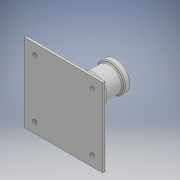
# Autodesk Inventor part: 相机
Saved by Autodesk Inventor 2017 (Build 210142000, 142)
## iProperties
Part Number: 相机
Material: 常规
Document SubType Name: Modeling
Designer: Administrator
Density: 1 g/cm^3
Appearance: 默认
Author: Administrator
Autodesk Inventor part; units mm, degrees
ref_plane "YZ Plane" through (0, 0, 0) normal (1, 0, 0) x (0, 1, 0)
ref_plane "XZ Plane" through (0, 0, 0) normal (0, 1, 0) x (-1, 0, 0)
ref_plane "XY Plane" through (0, 0, 0) normal (0, 0, 1) x (1, 0, 0)
sketch "草图1" plane through (0, 0, 0) normal (0, 1, 0) x (-1, 0, 0)
  line L0 (19, 19) -> (19, -19)
  line L1 (19, -19) -> (-19, -19)
  line L2 (-19, -19) -> (-19, 19)
  line L3 (-19, 19) -> (19, 19)
  line L4 (19, 19) -> (-19, -19) construction
  line L5 (19, -19) -> (-19, 19) construction
  line L6 (14, 14) -> (-14, -14) construction
  line L7 (14, -14) -> (-14, 14) construction
  circle A0 centre (14, 14) radius 1
  circle A1 centre (14, -14) radius 1
  circle A2 centre (-14, -14) radius 1
  circle A3 centre (-14, 14) radius 1
  line L8 (8, 8) -> (-8, -8) construction
  line L9 (8, -8) -> (-8, 8) construction
  point P0 (0, 0)
  dimension "d0" = 38
  dimension "d1" = 38
  dimension "d3" = 28
  dimension "d4" = 2
  dimension "d5" = 2
  dimension "d6" = 2
  dimension "d7" = 2
  constraints: 20 end point, 6 midpoint, 4 centre point, 4 coincident, 2 parallel, 1 perpendicular, 1 vertical
  measures "d0" distance of L0.start L0.end
  measures "d1" distance of L0.end L1.end
  measures "d3" distance of L7.start L6.end
  measures "d4" diameter of A0
  measures "d5" diameter of A1
  measures "d6" diameter of A2
  measures "d7" diameter of A3
extrude "拉伸1" add sketch "草图1" along normal blind 1.5
sketch "草图2" plane through (0, 1.5, 0) normal (0, 1, 0) x (1, 0, 0)
  line L0 (-8, -8) -> (-8, 8)
  line L1 (-8, 8) -> (8, 8)
  line L2 (8, 8) -> (8, -8)
  line L3 (8, -8) -> (-8, -8)
  line L4 (-8, -8) -> (8, 8) construction
  line L5 (-8, 8) -> (8, -8) construction
  point P0 (0, 0)
  dimension "d12" = 16
  dimension "d13" = 16
  constraints: 12 end point, 2 midpoint, 2 parallel, 1 perpendicular, 1 vertical
  measures "d12" distance of L0.start L0.end
  measures "d13" distance of L0.end L1.end
sketch "草图3" plane through (0, 1.5, 0) normal (0, 1, 0) x (1, 0, 0)
  point P0 (0, 0)
extrude "拉伸2" add sketch "草图2" along normal blind 4
sketch "草图4" plane through (0, 5.5, 0) normal (0, 1, 0) x (1, 0, 0)
  circle A0 centre (0, 0) radius 7
  dimension "d16" = 14
  constraints: 1 centre point, 1 coincident
  measures "d16" diameter of A0
extrude "拉伸3" add sketch "草图4" along normal blind 9
sketch "草图5" plane through (0, 14.5, 0) normal (0, 1, 0) x (1, 0, 0)
  circle A0 centre (0, 0) radius 6
  dimension "d19" = 12
  constraints: 1 centre point, 1 coincident
  measures "d19" diameter of A0
extrude "拉伸4" add sketch "草图5" along normal blind 8
sketch "草图6" plane through (0, 22.5, 0) normal (0, 1, 0) x (1, 0, 0)
  circle A0 centre (0, 0) radius 7
  dimension "d22" = 14
  constraints: 1 centre point, 1 coincident
  measures "d22" diameter of A0
extrude "拉伸5" add sketch "草图6" along normal blind 3
sketch "草图8" plane through (0, 25.5, 0) normal (0, 1, 0) x (1, 0, 0)
  circle A0 centre (0, 0) radius 6
  dimension "d29" = 12
  constraints: 1 centre point, 1 coincident
  measures "d29" diameter of A0
extrude "拉伸6" cut sketch "草图8" against normal blind 2
fillet "圆角1" radius 0.5 22 edges at (-7, 25.5, 0) (-7, 22.5, 0) (-6, 22.5, 0) (-6, 14.5, 0) (-7, 14.5, 0) (-7, 5.5, 0) (0, 5.5, 8) (8, 5.5, 0) (0, 5.5, -8) (-8, 5.5, 0) (19, 1.5, 0) (0, 1.5, 19) (-19, 1.5, 0) (0, 1.5, -19) (-8, 3.5, 8) (8, 3.5, 8) (-8, 3.5, -8) (-8, 1.5, 0) (0, 1.5, 8) (8, 1.5, 0) (8, 3.5, -8) (0, 1.5, -8)
